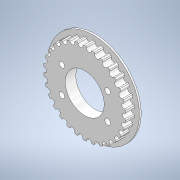
# Autodesk Inventor part: プーリ_歯数30
Saved by Autodesk Inventor 2021 (Build 250183000, 183)
## iProperties
Created: 2022-02-01
Part Number: プーリ_歯数30
Material: アセタール樹脂、白
Document SubType Name: Modeling
Designer: hirohumi
Density: 1.425 g/cm^3
Appearance: 滑らか - 白
Mass: 10.4181 g
Surface Area: 49.5548 cm^2
Volume: 7.31097 cm^3
Author: hirohumi
Autodesk Inventor part; units mm, degrees
ref_plane "YZ Plane" through (0, 0, 0) normal (1, 0, 0) x (0, 1, 0)
ref_plane "XZ Plane" through (0, 0, 0) normal (0, 1, 0) x (-1, 0, 0)
ref_plane "XY Plane" through (0, 0, 0) normal (0, 0, 1) x (1, 0, 0)
sketch "スケッチ1" plane through (0, 0, 0) normal (0, 0, 1) x (1, 0, 0)
  arc A0 (9.5012, 19.1434) -> (-9.5755, 19.1063) centre (0, 0) ccw construction
  arc A1 (8.6448, 22.2528) -> (-7.4379, 22.6848) centre (0, 0) ccw construction
  arc A2 (0.516, 23.2958) -> (-0.516, 23.2958) centre (0, 0) ccw
  arc A3 (-0.516, 23.2958) -> (-1.0127, 22.7401) centre (-0.5047, 22.7859) ccw
  arc A4 (1.0127, 22.7401) -> (0.516, 23.2958) centre (0.5047, 22.7859) ccw
  arc A5 (-2.2339, 21.2544) -> (-1.0127, 22.7401) centre (-2.3771, 22.6169) ccw
  arc A6 (1.0127, 22.7401) -> (2.2339, 21.2544) centre (2.3771, 22.6169) ccw
  line L0 (-2.2339, 21.2544) -> (0, 0)
  line L1 (0, 0) -> (2.2339, 21.2544)
  line L2 (0, 0) -> (0, 7.6483) construction
  dimension "d0" = 23.873
  dimension "d1" = 0.5715
  dimension "d2" = 0.51
  dimension "d3" = 0.51
  dimension "d4" = 1.37
  dimension "d5" = 1.37
  dimension "d6" = 1.93
  dimension "d7" = 12
  dimension "d8" = 6
  constraints: 16 point on circle, 7 centre point, 6 end point, 6 tangent, 3 coincident, 1 vertical
  measures "d0" radius of A1
  measures "d1" radial gap between concentric circles of A2 A1
  measures "d2" radius of A3
  measures "d3" radius of A4
  measures "d4" radius of A5
  measures "d5" radius of A6
  measures "d6" radial gap between concentric circles of A0 A2
  measures "d7" angle of L1 L0
  measures "d8" angle of L2 L0
extrude "押し出し1" add sketch "スケッチ1" along normal blind 5
pattern_circular "円形状パターン1" count 30 over 360 about axis through (0, 0, 0) along (0, 0, 1) of "押し出し1"
sketch "スケッチ2" plane through (0, 0, 0) normal (0, 0, -1) x (-1, 0, 0)
  circle A0 centre (0, 0) radius 26
  dimension "d14" = 52
  constraints: 1 centre point, 1 coincident
  measures "d14" diameter of A0
extrude "押し出し2" add sketch "スケッチ2" along normal blind 1
sketch "スケッチ3" plane through (0, 0, 5) normal (0, 0, 1) x (1, 0, 0)
  circle A0 centre (0, 0) radius 11.05
  circle A1 centre (0, 0) radius 15 construction
  circle A2 centre (-12.9904, 7.5) radius 1.6
  circle A3 centre (-12.9904, -7.5) radius 1.6
  circle A4 centre (12.9904, -7.5) radius 1.6
  circle A5 centre (12.9904, 7.5) radius 1.6
  dimension "d17" = 22.1
  dimension "d18" = 30
  dimension "d19" = 3.2
  dimension "d20" = 3.2
  dimension "d21" = 3.2
  dimension "d22" = 3.2
  dimension "d23" = 15
  dimension "d24" = 7.5
  constraints: 6 centre point, 4 point on circle, 2 coincident, 2 horizontal alignment
  measures "d17" diameter of A0
  measures "d18" diameter of A1
  measures "d19" diameter of A2
  measures "d20" diameter of A3
  measures "d21" diameter of A4
  measures "d22" diameter of A5
  measures "d23" distance of A3.centre A2.centre
  measures "d24" vertical distance of point (0, 0) A3.centre
extrude "押し出し3" cut sketch "スケッチ3" against normal through all
